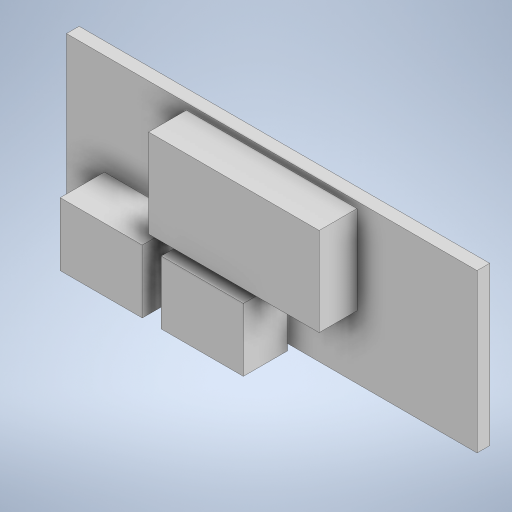
# Autodesk Inventor part: Power
Saved by Autodesk Inventor 2024 (Build 280153000, 153)
## iProperties
Created: 2024-03-12
Part Number: Power
Material: Générique
Document SubType Name: Modeling
Designer: phaly
Density: 1 g/cm^3
Appearance: Par défaut
Author: phaly
Autodesk Inventor part; units mm, degrees
ref_plane "YZ Plane" through (0, 0, 0) normal (1, 0, 0) x (0, 1, 0)
ref_plane "XZ Plane" through (0, 0, 0) normal (0, 1, 0) x (-1, 0, 0)
ref_plane "XY Plane" through (0, 0, 0) normal (0, 0, 1) x (1, 0, 0)
sketch "Esquisse1" plane through (0, 0, 0) normal (0, 0, 1) x (1, 0, 0)
  line L0 (0, 25) -> (65, 25)
  line L1 (65, 25) -> (65, 0)
  line L2 (65, 0) -> (0, 0)
  line L3 (0, 0) -> (0, 25)
  line L4 (-13, 0) -> (78, 0) projected
  line L5 (0, -5) -> (0, 30) projected
  point P0 (0, 0)
  dimension "d0" = 25
  dimension "d1" = 65
  constraints: 8 end point, 2 collinear, 2 parallel, 1 horizontal, 1 perpendicular
  measures "d0" distance of L0.end L1.end
  measures "d1" distance of L0.start L0.end
extrude "Extrusion1" add sketch "Esquisse1" along normal blind 2
sketch "Esquisse2" plane through (0, 0, 2) normal (0, 0, 1) x (1, 0, 0)
  line L0 (19, 24) -> (46, 24)
  line L1 (46, 24) -> (46, 10)
  line L2 (46, 10) -> (19, 10)
  line L3 (19, 10) -> (19, 24)
  line L4 (65, 0) -> (65, 25) projected
  line L5 (65, 25) -> (0, 25) projected
  line L6 (0, 0) -> (65, 0) projected
  dimension "d4" = 27
  dimension "d6" = 19
  dimension "d11" = 10
  dimension "d12" = 1
  constraints: 8 end point, 2 parallel, 1 horizontal, 1 perpendicular
  measures "d4" distance of L0.start L0.end
  measures "d6" distance between parallel lines of L4 L1
  measures "d11" distance between parallel lines of L6 L2
  measures "d12" distance between parallel lines of L5 L0
extrude "Extrusion2" add sketch "Esquisse2" along normal blind 6
sketch "Esquisse3" plane through (0, 0, 2) normal (0, 0, 1) x (1, 0, 0)
  line L0 (6, 9) -> (19, 9)
  line L1 (19, 9) -> (19, -1)
  line L2 (19, -1) -> (6, -1)
  line L3 (6, -1) -> (6, 9)
  line L4 (0, 25) -> (0, 0) projected
  line L5 (0, 0) -> (65, 0) projected
  line L6 (22, 9) -> (35, 9)
  line L7 (35, 9) -> (35, -1)
  line L8 (35, -1) -> (22, -1)
  line L9 (22, -1) -> (22, 9)
  dimension "d10" = 10
  dimension "d13" = 13
  dimension "d14" = 6
  dimension "d15" = 1
  dimension "d16" = 10
  dimension "d17" = 13
  dimension "d18" = 3
  dimension "d19" = 1
  constraints: 16 end point, 4 parallel, 2 horizontal, 2 perpendicular
  measures "d10" distance of L2.end L0.start
  measures "d13" distance of L0.start L0.end
  measures "d14" distance between parallel lines of L4 L3
  measures "d15" distance between parallel lines of L5 L2
  measures "d16" distance of L8.end L6.start
  measures "d17" distance of L7.end L8.end
  measures "d18" distance between parallel lines of L1 L9
  measures "d19" distance between parallel lines of L5 L8
extrude "Extrusion3" add sketch "Esquisse3" along normal blind 7
equation "\"d16\" = d10"
equation "\"d17\" = d13"
equation "\"d19\" = d15"
